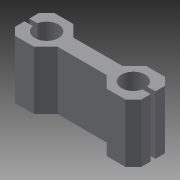
# Autodesk Inventor part: ChimeraXCarriage1
Saved by Autodesk Inventor 2015 (Build 190159000, 159)
## iProperties
Created: 2014-11-30
Part Number: ChimeraXCarriage1
Material: Generic
Document SubType Name: Modeling
Designer: Jack
Density: 1 g/cm^3
Appearance: Default
Author: Jack
Autodesk Inventor part; units mm, degrees
ref_plane "YZ Plane" through (0, 0, 0) normal (1, 0, 0) x (0, 1, 0)
ref_plane "XZ Plane" through (0, 0, 0) normal (0, 1, 0) x (-1, 0, 0)
ref_plane "XY Plane" through (0, 0, 0) normal (0, 0, 1) x (1, 0, 0)
sketch "Sketch2" plane through (0, 0, 0) normal (0, 0, 1) x (1, 0, 0)
  arc A0 (-7.3485, -1.5) -> (-7.3485, 1.5) centre (0, 0) ccw
  arc A1 (62.3485, 1.5) -> (62.3485, -1.5) centre (55, 0) ccw
  line L0 (-12.5, 12.5) -> (67.5, 12.5)
  line L1 (67.5, 12.5) -> (67.5, 1.5)
  line L2 (67.5, 1.5) -> (62.3485, 1.5)
  line L3 (62.3485, -1.5) -> (67.5, -1.5)
  line L4 (67.5, -1.5) -> (67.5, -12.5)
  line L5 (67.5, -12.5) -> (-12.5, -12.5)
  line L6 (-12.5, -12.5) -> (-12.5, -1.5)
  line L7 (-12.5, -1.5) -> (-7.3485, -1.5)
  line L8 (-7.3485, 1.5) -> (-12.5, 1.5)
  line L9 (-12.5, 1.5) -> (-12.5, 12.5)
  dimension "d17" = 15
  dimension "d18" = 55
  dimension "d20" = 3
  dimension "d21" = 1.5
  dimension "d22" = 12.5
  dimension "d23" = 12.5
  dimension "d24" = 12.5
  constraints: 20 end point, 6 perpendicular, 4 point on circle, 3 horizontal alignment, 3 point on line, 2 centre point, 2 parallel, 1 coincident, 1 collinear, 1 equal radius, 1 horizontal
  measures "d17" diameter of A0
  measures "d18" distance of A1.centre point (0, 0)
  measures "d20" distance between parallel lines of L8 L7
  measures "d21" distance from line of point (0, 0) L7
  measures "d22" distance from line of point (0, 0) L0
  measures "d23" distance from line of L5 point (0, 0)
  measures "d24" distance from line of point (0, 0) L9
extrude "Extrusion2" add sketch "Sketch2" along normal blind 37
chamfer "Chamfer1" distance 5 angle 45 4 edges at (-12.5, 12.5, 18.5) (-12.5, -12.5, 18.5) (67.5, 12.5, 18.5) (67.5, -12.5, 18.5)
sketch "Sketch3" plane through (0, 0, 37) normal (0, 0, 1) x (1, 0, 0)
  arc A0 (62.3485, 1.5) -> (62.3485, -1.5) centre (55, 0) ccw projected
  line L0 (62.5, 12.5) -> (-7.5, 12.5) projected
  arc A1 (-7.3485, -1.5) -> (-7.3485, 1.5) centre (0, 0) ccw projected
  line L1 (-7.5, -12.5) -> (62.5, -12.5) projected
  line L2 (4.5, 12.5) -> (12, 5)
  line L3 (12, 5) -> (43, 5)
  line L4 (43, 5) -> (50.5, 12.5)
  line L5 (4.5, -12.5) -> (12, -5)
  line L6 (12, -5) -> (43, -5)
  line L7 (43, -5) -> (50.5, -12.5)
  dimension "d30" = 135
  dimension "d31" = 10
  dimension "d32" = 135
  dimension "d33" = 12
  dimension "d34" = 12
  constraints: 12 end point, 4 point on line, 3 perpendicular, 2 vertical alignment, 1 horizontal, 1 parallel
  measures "d30" angle of L0 L2
  measures "d31" distance between parallel lines of L6 L3
  measures "d32" angle of L0 L4
  measures "d33" horizontal distance of A0.centre L3.end
  measures "d34" horizontal distance of A1.centre L2.end
extrude "Extrusion3" cut sketch "Sketch3" against normal up to next
body "Solid2"
